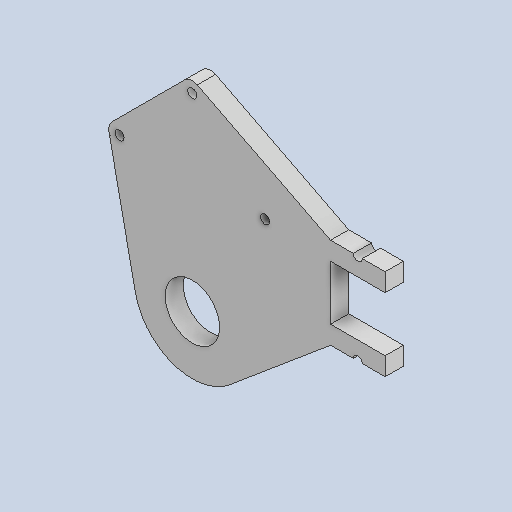
# Autodesk Inventor part: light_plate_nomo
Saved by Autodesk Inventor 2025.2 (Build 292293000, 293)
## iProperties
Created: 2025-05-05
Part Number: light_plate_nomo
Material: 一般
Document SubType Name: Modeling
Designer: yuki0520
Density: 1 g/cm^3
Appearance: 既定
Author: yuki0520
Autodesk Inventor part; units mm, degrees
ref_plane "YZ Plane" through (0, 0, 0) normal (1, 0, 0) x (0, 1, 0)
ref_plane "XZ Plane" through (0, 0, 0) normal (0, 1, 0) x (-1, 0, 0)
ref_plane "XY Plane" through (0, 0, 0) normal (0, 0, 1) x (1, 0, 0)
derived "zzz_light_plate.ipt"
sketch "スケッチ1" plane through (0, 0, 0) normal (0, 0, 1) x (1, 0, 0)
  circle A0 centre (0, 0) radius 120
  line L0 (12.25, 120) -> (-12.25, 120)
  line L1 (-12.25, 120) -> (-12.25, 196)
  line L2 (-12.25, 196) -> (12.25, 196)
  line L3 (12.25, 196) -> (12.25, 120)
  line L4 (12.25, 120) -> (-12.25, 196) construction
  line L5 (-12.25, 120) -> (12.25, 196) construction
  line L6 (-41.25, 158) -> (95.75, 158)
  line L7 (0, -120) -> (0, 120)
  line L8 (59.75, 218) -> (59.75, 138)
  circle A1 centre (400, 0) radius 120
  circle A2 centre (400, 158) radius 38
  line L9 (400, -120) -> (400, 120)
  line L10 (-120, 0) -> (120, 0)
  circle A3 centre (400, 158) radius 16
  circle A4 centre (400, 190) radius 16
  circle A5 centre (400, 190) radius 12
  line L11 (102.75, 178) -> (59.75, 178)
  line L12 (59.75, 178) -> (59.75, 202)
  line L13 (59.75, 202) -> (102.75, 202)
  line L14 (102.75, 202) -> (102.75, 178)
  line L15 (102.75, 178) -> (59.75, 202) construction
  line L16 (59.75, 178) -> (102.75, 202) construction
  line L17 (57.75, 218) -> (57.75, 121.8661)
  circle A6 centre (400, 190) radius 9.5
  circle A7 centre (400, 190) radius 6.55
  circle A8 centre (404.3332, 198.4542) radius 1.3
  circle A9 centre (390.5119, 189.5255) radius 1.3
  circle A10 centre (405.155, 182.0203) radius 1.3
  line L18 (135, 218) -> (-135, 218)
  line L19 (-135, 218) -> (-135, 203)
  line L20 (-135, 203) -> (135, 203)
  line L21 (135, 203) -> (135, 218)
  circle A11 centre (400, 158) radius 7.5
  line L22 (-35.25, 218) -> (-35.25, 138)
  line L23 (22.25, 218) -> (22.25, 138)
  line L24 (17.25, 138) -> (17.25, 218)
  line L25 (-30.25, 218) -> (-30.25, 138)
  line L26 (12.25, -196) -> (12.25, -120)
  line L27 (12.25, -120) -> (-12.25, -196) construction
  line L28 (-12.25, -120) -> (-12.25, -196)
  line L29 (12.25, -120) -> (-12.25, -120)
  line L30 (-12.25, -120) -> (12.25, -196) construction
  line L31 (-12.25, -196) -> (12.25, -196)
  line L32 (17.25, -138) -> (17.25, -218)
  line L33 (-41.25, -158) -> (95.75, -158)
  line L34 (-135, -203) -> (135, -203)
  line L35 (135, -218) -> (-135, -218)
  line L36 (57.75, -218) -> (57.75, -121.8661)
  line L37 (135, -203) -> (135, -218)
  line L38 (59.75, -218) -> (59.75, -138)
  line L39 (22.25, -218) -> (22.25, -138)
  line L40 (59.75, -178) -> (59.75, -202)
  line L41 (102.75, -178) -> (59.75, -178)
  line L42 (102.75, -178) -> (59.75, -202) construction
  line L43 (102.75, -202) -> (102.75, -178)
  line L44 (59.75, -178) -> (102.75, -202) construction
  line L45 (-35.25, -218) -> (-35.25, -138)
  line L46 (-135, -218) -> (-135, -203)
  line L47 (-30.25, -218) -> (-30.25, -138)
  line L48 (46.75, -182) -> (56.75, -182)
  line L49 (60, -182) -> (50, -182)
  line L50 (59.75, -202) -> (102.75, -202)
  line L51 (46.75, -134) -> (56.75, -182) construction
  line L52 (56.75, -134) -> (46.75, -134)
  line L53 (56.75, -182) -> (56.75, -134)
  line L54 (46.75, -134) -> (46.75, -182)
  line L55 (56.75, -134) -> (46.75, -182) construction
  line L56 (-135, 203) -> (-135, -203)
  line L57 (453, 189) -> (438, 189)
  line L58 (438, 189) -> (438, 174)
  line L59 (438, 174) -> (453, 174)
  line L60 (453, 174) -> (453, 189)
  line L61 (438, 158) -> (438, -0.316)
  circle A12 centre (480, 0) radius 120
  line L62 (605, 50) -> (600, 50)
  line L63 (600, 50) -> (600, -50)
  line L64 (600, -50) -> (605, -50)
  line L65 (605, -50) -> (605, 50)
  line L66 (438, 174) -> (453, 174)
  line L67 (453, 174) -> (453, 169)
  line L68 (453, 169) -> (438, 169)
  line L69 (438, 169) -> (438, 174)
  arc A13 (600, 50) -> (453, 169) centre (359.7884, -96.4378) ccw
  line L70 (438, 189) -> (453, 189)
  line L71 (453, 189) -> (453, 194)
  line L72 (453, 194) -> (438, 194)
  line L73 (438, 194) -> (438, 189)
  arc A14 (605, 50) -> (453, 194) centre (369.2063, -46.6712) ccw
  circle A15 centre (400, 136.2498) radius 38
  circle A16 centre (420, 190) radius 3
  circle A17 centre (400, 190) radius 20
  circle A18 centre (400, 210) radius 3
  circle A19 centre (380, 190) radius 3
  line L74 (438, 169) -> (410.2848, 145.7434)
  line L75 (438, 194) -> (401.3623, 212.6729)
  line L76 (397.8787, 212.1213) -> (377.8787, 192.1213)
  line L77 (384.3412, 154.7133) -> (377.064, 189.3837)
  circle A20 centre (420, 190) radius 1.25
  circle A21 centre (400, 210) radius 1.25
  circle A22 centre (380, 190) radius 1.25
  circle A23 centre (445.5, 194) radius 1.25
  circle A24 centre (445.5, 169) radius 1.25
  line L78 (57.75, 193) -> (40.75, 193)
  line L79 (40.75, 193) -> (40.75, 187)
  line L80 (40.75, 187) -> (57.75, 187)
  line L81 (57.75, 187) -> (57.75, 193)
  line L82 (102.75, 190) -> (81.25, 190)
  line L83 (22.25, 167) -> (23.25, 167)
  line L84 (23.25, 167) -> (23.25, 149)
  line L85 (23.25, 149) -> (22.25, 149)
  line L86 (22.25, 149) -> (22.25, 167)
  line L87 (23.25, 166.5) -> (30.75, 166.5)
  line L88 (30.75, 166.5) -> (30.75, 149.5)
  line L89 (30.75, 149.5) -> (23.25, 149.5)
  line L90 (23.25, 149.5) -> (23.25, 166.5)
  line L91 (37.75, 174) -> (42.75, 174)
  line L92 (42.75, 174) -> (42.75, 142)
  line L93 (42.75, 142) -> (37.75, 142)
  line L94 (37.75, 142) -> (37.75, 174)
  line L95 (37.75, 174) -> (42.75, 174)
  line L96 (42.75, 174) -> (42.75, 206)
  line L97 (42.75, 206) -> (37.75, 206)
  line L98 (37.75, 206) -> (37.75, 174)
  line L99 (37.75, 190) -> (42.75, 190)
  line L100 (42.75, 200) -> (52.75, 200)
  line L101 (52.75, 200) -> (52.75, 180)
  line L102 (52.75, 180) -> (42.75, 180)
  line L103 (42.75, 180) -> (42.75, 200)
  point P0 (0, 158)
  point P1 (0, -158)
  point P2 (51.75, -158)
  point P3 (65.8106, -158)
  point P4 (446.75, 194)
  point P5 (444.25, 194)
  point P6 (377.3818, 188.5355)
  point P7 (377.2609, 188.4456)
  point P8 (444.25, 169)
  point P9 (446.75, 169)
  dimension "d22" = 2.5
  dimension "d23" = 2.5
  dimension "d24" = 2.5
  dimension "d25" = 2.5
  dimension "d26" = 2.5
  measures "d22" diameter of A20
  measures "d23" diameter of A21
  measures "d24" diameter of A22
  measures "d25" diameter of A23
  measures "d26" diameter of A24
extrude "押し出し4" add sketch "スケッチ1" against normal blind 5 contours L68 A24 L69 L59 L67 | L74 A15 A17 A16 A2 | A2 A16 A17 A18 L75 L73 L58 L69 L74 | L74 A3 A17 A15 | L71 L57 L73 L72 A23 | A2 A19 A17 A15 L77 | A15 A17 A3 L77 | A16 A17 A20 A2 | A2 A20 A17 A16 | A17 A3 A4 A15 | A15 A4 A2 A16 A17 | A3 A17 | A19 A17 A22 A2 | A2 A22 A17 A19 | A17 A19 A2 A4 A15 | A15 A4 A3 A17 | A16 A2 A20 A17 | A15 A4 A2 A5 | A4 A15 | A17 A3 | A17 A22 A2 A19 | L76 A17 A19 | A16 A17 A20 A2 | A2 A4 A19 A17 L76 A18 A16 | A17 A19 A2 A22 | A4 A2 A5 | A18 A17 A21 | A17 A21 A18 | L76 A18 A17 | A5 A2 A6 A8 | A2 A6 A9 A10 A5 | A6 A8 A2 A7 | A2 A7 A6 A10 A9 | A7 A2 | A2 A7 | A8 A6 | A6 A8 | A9 A6 | A6 A9 | A10 A6 | A6 A10
